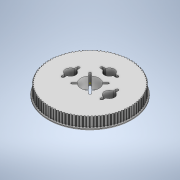
# Autodesk Inventor part: ZebatkaSilnik3
Saved by Autodesk Inventor 2021 (Build 250183000, 183)
## iProperties
Created: 2021-03-23
Part Number: ZebatkaSilnik3
Material: Ogólny
Document SubType Name: Modeling
Designer: micha
Density: 1 g/cm^3
Appearance: Domyślna
Author: micha
Autodesk Inventor part; units mm, degrees
(part 1 of 2)
ref_plane "YZ Plane" through (0, 0, 0) normal (1, 0, 0) x (0, 1, 0)
ref_plane "XZ Plane" through (0, 0, 0) normal (0, 1, 0) x (-1, 0, 0)
ref_plane "XY Plane" through (0, 0, 0) normal (0, 0, 1) x (1, 0, 0)
sketch "Szkic1" plane through (0, 0, 0) normal (0, 1, 0) x (-1, 0, 0)
  circle A0 centre (0, 0) radius 32.5
  dimension "d0" = 65
  constraints: 1 centre point, 1 coincident
  measures "d0" diameter of A0
extrude "Wyciągnięcie proste1" add sketch "Szkic1" along normal blind 1.5
sketch "Szkic3" plane through (0, 1.5, 0) normal (0, 1, 0) x (1, 0, 0)
  circle A0 centre (0, 0) radius 32.5 projected
  arc A1 (-30.7875, -0.0069) -> (-31.0611, 0.5149) centre (-31.3409, 0.0356) ccw
  arc A2 (-31.0611, 0.5149) -> (-31.3613, 0.6303) centre (-31.5652, -0.3487) ccw
  arc A3 (-31.4793, 0.7983) -> (-31.3613, 0.6303) centre (-31.3308, 0.7772) ccw
  line L0 (-32.4607, 1.0462) -> (-32.4793, 0.7969)
  line L1 (-31.4606, -1.0449) -> (-31.4793, -0.7955)
  arc A4 (-31.3613, -0.6278) -> (-31.4793, -0.7955) centre (-31.3307, -0.7746) ccw
  arc A5 (-31.061, -0.5126) -> (-30.7873, 0.0071) centre (-31.3409, -0.0332) ccw
  arc A6 (-31.3613, -0.6278) -> (-31.061, -0.5126) centre (-31.5647, 0.3513) ccw
  circle A7 centre (0, 0) radius 31.5
  line L2 (-31.4606, 1.0476) -> (-31.4793, 0.7983)
  line L3 (-31.3329, -3.0182) -> (-31.3672, -2.7706)
  arc A8 (-31.26, -2.5957) -> (-31.3672, -2.7706) centre (-31.2203, -2.7404) ccw
  arc A9 (-31.26, -2.5957) -> (-30.9676, -2.4619) centre (-31.5245, -1.6313) ccw
  arc A10 (-30.9676, -2.4619) -> (-30.727, -1.9261) centre (-31.2769, -2.0011) ccw
  arc A11 (-30.7263, -1.9401) -> (-31.0321, -1.4364) centre (-31.2813, -1.9323) ccw
  arc A12 (-31.0321, -1.4364) -> (-31.339, -1.3401) centre (-31.481, -2.33) ccw
  arc A13 (-31.4673, -1.1799) -> (-31.339, -1.3401) centre (-31.3177, -1.1916) ccw
  line L4 (-31.4643, -0.9299) -> (-31.4673, -1.1799)
  circle A14 centre (0, 0) radius 31.5
  line L5 (-31.0816, -4.9797) -> (-31.1313, -4.7347)
  arc A15 (-31.0354, -4.5534) -> (-31.1313, -4.7347) centre (-30.9866, -4.6953) ccw
  arc A16 (-31.0354, -4.5534) -> (-30.7519, -4.4015) centre (-31.3599, -3.6075) ccw
  arc A17 (-30.7519, -4.4015) -> (-30.5454, -3.8516) centre (-31.0896, -3.961) ccw
  arc A18 (-30.5439, -3.8656) -> (-30.8807, -3.3821) centre (-31.0982, -3.8927) ccw
  arc A19 (-30.8807, -3.3821) -> (-31.193, -3.3053) centre (-31.2726, -4.3021) ccw
  arc A20 (-31.3311, -3.1534) -> (-31.193, -3.3053) centre (-31.1811, -3.1557) ccw
  line L6 (-31.3438, -2.9037) -> (-31.3311, -3.1534)
  circle A21 centre (0, 0) radius 31.5
  line L7 (-30.7076, -6.9215) -> (-30.7726, -6.6801)
  arc A22 (-30.6882, -6.4932) -> (-30.7726, -6.6801) centre (-30.6306, -6.6317) ccw
  arc A23 (-30.6882, -6.4932) -> (-30.4148, -6.3237) centre (-31.0715, -5.5695) ccw
  arc A24 (-30.4148, -6.3237) -> (-30.2433, -5.762) centre (-30.7795, -5.9054) ccw
  arc A25 (-30.2409, -5.7758) -> (-30.6074, -5.3144) centre (-30.7924, -5.8377) ccw
  arc A26 (-30.6074, -5.3144) -> (-30.924, -5.2574) centre (-30.9408, -6.2572) ccw
  arc A27 (-31.0713, -5.1145) -> (-30.924, -5.2574) centre (-30.9214, -5.1074) ccw
  line L8 (-31.0996, -4.8661) -> (-31.0713, -5.1145)
  circle A28 centre (0, 0) radius 31.5
  line L9 (-30.2124, -8.836) -> (-30.2924, -8.5991)
  arc A29 (-30.2199, -8.4073) -> (-30.2924, -8.5991) centre (-30.1538, -8.5419) ccw
  arc A30 (-30.2199, -8.4073) -> (-29.9577, -8.221) centre (-30.6604, -7.5095) ccw
  arc A31 (-29.9577, -8.221) -> (-29.8219, -7.6496) centre (-30.348, -7.8264) ccw
  arc A32 (-29.8185, -7.6633) -> (-30.2133, -7.2258) centre (-30.3651, -7.7596) ccw
  arc A33 (-30.2133, -7.2258) -> (-30.5328, -7.1887) centre (-30.4868, -8.1877) ccw
  arc A34 (-30.6888, -7.0554) -> (-30.5328, -7.1887) centre (-30.5397, -7.0389) ccw
  line L10 (-30.7327, -6.8093) -> (-30.6888, -7.0554)
  circle A35 centre (0, 0) radius 31.5
  line L11 (-29.5979, -10.7156) -> (-29.6927, -10.4842)
  arc A36 (-29.6324, -10.2882) -> (-29.6927, -10.4842) centre (-29.5579, -10.4184) ccw
  arc A37 (-29.6324, -10.2882) -> (-29.3824, -10.0859) centre (-30.1284, -9.4199) ccw
  arc A38 (-29.3824, -10.0859) -> (-29.2827, -9.507) centre (-29.7966, -9.7165) ccw
  arc A39 (-29.2785, -9.5205) -> (-29.7, -9.1087) centre (-29.818, -9.651) ccw
  arc A40 (-29.7, -9.1087) -> (-30.0212, -9.0917) centre (-29.9126, -10.0858) ccw
  arc A41 (-30.1853, -8.9684) -> (-30.0212, -9.0917) centre (-30.0375, -8.9426) ccw
  line L12 (-30.2445, -8.7255) -> (-30.1853, -8.9684)
  circle A42 centre (0, 0) radius 31.5
  line L13 (-28.8667, -12.5529) -> (-28.9758, -12.328)
  arc A43 (-28.9279, -12.1285) -> (-28.9758, -12.328) centre (-28.8454, -12.2538) ccw
  arc A44 (-28.9279, -12.1285) -> (-28.6911, -11.9109) centre (-29.4775, -11.2931) ccw
  arc A45 (-28.6911, -11.9109) -> (-28.6279, -11.327) centre (-29.1277, -11.5683) ccw
  arc A46 (-28.623, -11.3401) -> (-29.0694, -10.9556) centre (-29.1531, -11.5042) ccw
  arc A47 (-29.0694, -10.9556) -> (-29.3911, -10.9588) centre (-29.2203, -11.9441) ccw
  arc A48 (-29.5626, -10.8461) -> (-29.3911, -10.9588) centre (-29.4167, -10.811) ccw
  line L14 (-29.637, -10.6074) -> (-29.5626, -10.8461)
  circle A49 centre (0, 0) radius 31.5
  line L15 (-28.0215, -14.3407) -> (-28.1446, -14.1231)
  arc A50 (-28.1093, -13.921) -> (-28.1446, -14.1231) centre (-28.0191, -14.0409) ccw
  arc A51 (-28.1093, -13.921) -> (-27.8866, -13.6889) centre (-28.7102, -13.1217) ccw
  arc A52 (-27.8866, -13.6889) -> (-27.8602, -13.1022) centre (-28.3439, -13.3744) ccw
  arc A53 (-27.8544, -13.115) -> (-28.3242, -12.7592) centre (-28.3732, -13.312) ccw
  arc A54 (-28.3242, -12.7592) -> (-28.645, -12.7827) centre (-28.4126, -13.7553) ccw
  arc A55 (-28.8232, -12.6809) -> (-28.645, -12.7827) centre (-28.6798, -12.6368) ccw
  line L16 (-28.9124, -12.4474) -> (-28.8232, -12.6809)
  circle A56 centre (0, 0) radius 31.5
  line L17 (-27.0658, -16.0719) -> (-27.2022, -15.8624)
  arc A57 (-27.1797, -15.6585) -> (-27.2022, -15.8624) centre (-27.0822, -15.7725) ccw
  arc A58 (-27.1797, -15.6585) -> (-26.9721, -15.4129) centre (-27.8296, -14.8985) ccw
  arc A59 (-26.9721, -15.4129) -> (-26.9826, -14.8257) centre (-27.4482, -15.1277) ccw
  arc A60 (-26.976, -14.8381) -> (-27.4671, -14.5125) centre (-27.4814, -15.0674) ccw
  arc A61 (-27.4671, -14.5125) -> (-27.7858, -14.5561) centre (-27.4928, -15.5122) ccw
  arc A62 (-27.9701, -14.4657) -> (-27.7858, -14.5561) centre (-27.8298, -14.4127) ccw
  line L18 (-28.0738, -14.2382) -> (-27.9701, -14.4657)
  circle A63 centre (0, 0) radius 31.5
  line L19 (-26.0032, -17.7396) -> (-26.1526, -17.5391)
  arc A64 (-26.1429, -17.3343) -> (-26.1526, -17.5391) centre (-26.0384, -17.4419) ccw
  arc A65 (-26.1429, -17.3343) -> (-25.9511, -17.0761) centre (-26.8392, -16.6166) ccw
  arc A66 (-25.9511, -17.0761) -> (-25.9984, -16.4907) centre (-26.4441, -16.8213) ccw
  arc A67 (-25.991, -16.5026) -> (-26.5017, -16.2086) centre (-26.4811, -16.7632) ccw
  arc A68 (-26.5017, -16.2086) -> (-26.817, -16.272) centre (-26.4646, -17.2079) ccw
  arc A69 (-27.0066, -16.1934) -> (-26.817, -16.272) centre (-26.8699, -16.1317) ccw
  line L20 (-27.1244, -15.9729) -> (-27.0066, -16.1934)
  circle A70 centre (0, 0) radius 31.5
  line L21 (-24.838, -19.3374) -> (-24.9997, -19.1467)
  arc A71 (-25.0029, -18.9416) -> (-24.9997, -19.1467) centre (-24.8918, -19.0424) ccw
  arc A72 (-25.0029, -18.9416) -> (-24.8276, -18.6719) centre (-25.7429, -18.269) ccw
  arc A73 (-24.8276, -18.6719) -> (-24.9117, -18.0906) centre (-25.3357, -18.4486) ccw
  arc A74 (-24.9035, -18.1021) -> (-25.4316, -17.8406) centre (-25.3763, -18.3929) ccw
  arc A75 (-25.4316, -17.8406) -> (-25.7424, -17.9238) centre (-25.3319, -18.8357) ccw
  arc A76 (-25.9365, -17.8572) -> (-25.7424, -17.9238) centre (-25.8039, -17.787) ccw
  line L22 (-26.0679, -17.6446) -> (-25.9365, -17.8572)
  circle A77 centre (0, 0) radius 31.5
  line L23 (-23.5748, -20.8588) -> (-23.7481, -20.6786)
  arc A78 (-23.7642, -20.4742) -> (-23.7481, -20.6786) centre (-23.647, -20.5678) ccw
  arc A79 (-23.7642, -20.4742) -> (-23.6062, -20.194) centre (-24.545, -19.8494) ccw
  arc A80 (-23.6062, -20.194) -> (-23.7266, -19.6191) centre (-24.1273, -20.003) ccw
  arc A81 (-23.7178, -19.6301) -> (-24.2612, -19.4023) centre (-24.1713, -19.95) ccw
  arc A82 (-24.2612, -19.4023) -> (-24.5661, -19.5048) centre (-24.0992, -20.3891) ccw
  arc A83 (-24.764, -19.4506) -> (-24.5661, -19.5048) centre (-24.6362, -19.3722) ccw
  line L24 (-24.9086, -19.2466) -> (-24.764, -19.4506)
  circle A84 centre (0, 0) radius 31.5
  line L25 (-22.2185, -22.2979) -> (-22.4028, -22.129)
  arc A85 (-22.4317, -21.9259) -> (-22.4028, -22.129) centre (-22.3089, -22.012) ccw
  arc A86 (-22.4317, -21.9259) -> (-22.2917, -21.6364) centre (-23.2502, -21.3514) ccw
  arc A87 (-22.2917, -21.6364) -> (-22.4479, -21.0702) centre (-22.8237, -21.4785) ccw
  arc A88 (-22.4384, -21.0806) -> (-22.9951, -20.8874) centre (-22.8709, -21.4283) ccw
  arc A89 (-22.9951, -20.8874) -> (-23.2929, -21.0088) centre (-22.7714, -21.8621) ccw
  arc A90 (-23.4939, -20.9671) -> (-23.2929, -21.0088) centre (-23.3712, -20.8808) ccw
  line L26 (-23.6509, -20.7726) -> (-23.4939, -20.9671)
  circle A91 centre (0, 0) radius 31.5
  line L27 (-20.7746, -23.649) -> (-20.9691, -23.492)
  arc A92 (-21.0107, -23.2912) -> (-20.9691, -23.492) centre (-20.8827, -23.3694) ccw
  arc A93 (-21.0107, -23.2912) -> (-20.8891, -22.9934) centre (-21.8637, -22.7692) ccw
  arc A94 (-20.8891, -22.9934) -> (-21.0806, -22.4381) centre (-21.4301, -22.8693) ccw
  arc A95 (-21.0704, -22.4479) -> (-21.6382, -22.29) centre (-21.4803, -22.8221) ccw
  arc A96 (-21.6382, -22.29) -> (-21.9278, -22.4299) centre (-21.3537, -23.2487) ccw
  arc A97 (-22.131, -22.4009) -> (-21.9278, -22.4299) centre (-22.0139, -22.3071) ccw
  line L28 (-22.2999, -22.2167) -> (-22.131, -22.4009)
  circle A98 centre (0, 0) radius 31.5
  line L29 (-19.2487, -24.9068) -> (-19.4527, -24.7623)
  arc A99 (-19.5068, -24.5645) -> (-19.4527, -24.7623) centre (-19.3741, -24.6345) ccw
  arc A100 (-19.5068, -24.5645) -> (-19.4041, -24.2597) centre (-20.3908, -24.0971) ccw
  arc A101 (-19.4041, -24.2597) -> (-19.6301, -23.7175) centre (-19.9518, -24.1697) ccw
  arc A102 (-19.6193, -23.7266) -> (-20.1958, -23.6047) centre (-20.0049, -24.1258) ccw
  arc A103 (-20.1958, -23.6047) -> (-20.4761, -23.7625) centre (-19.8518, -24.5437) ccw
  arc A104 (-20.6807, -23.7463) -> (-20.4761, -23.7625) centre (-20.5698, -23.6454) ccw
  line L30 (-20.8609, -23.573) -> (-20.6807, -23.7463)
  circle A105 centre (0, 0) radius 31.5
  line L31 (-17.6468, -26.0663) -> (-17.8594, -25.9349)
  arc A106 (-17.9259, -25.7408) -> (-17.8594, -25.9349) centre (-17.7891, -25.8024) ccw
  arc A107 (-17.9259, -25.7408) -> (-17.8426, -25.4302) centre (-18.8375, -25.3299) ccw
  arc A108 (-17.8426, -25.4302) -> (-18.1021, -24.9033) centre (-18.3948, -25.3748) ccw
  arc A109 (-18.0908, -24.9117) -> (-18.6738, -24.8263) centre (-18.4505, -25.3344) ccw
  arc A110 (-18.6738, -24.8263) -> (-18.9437, -25.0014) centre (-18.2715, -25.7417) ccw
  arc A111 (-19.1489, -24.998) -> (-18.9437, -25.0014) centre (-19.0445, -24.8903) ccw
  line L32 (-19.3396, -24.8364) -> (-19.1489, -24.998)
  circle A112 centre (0, 0) radius 31.5
  line L33 (-15.9752, -27.1229) -> (-16.1957, -27.0051)
  arc A113 (-16.2742, -26.8156) -> (-16.1957, -27.0051) centre (-16.1338, -26.8685) ccw
  arc A114 (-16.2742, -26.8156) -> (-16.2106, -26.5004) centre (-17.2099, -26.4627) ccw
  arc A115 (-16.2106, -26.5004) -> (-16.5027, -25.9908) centre (-16.7652, -26.4798) ccw
  arc A116 (-16.4909, -25.9985) -> (-17.0781, -25.9498) centre (-16.8234, -26.4429) ccw
  arc A117 (-17.0781, -25.9498) -> (-17.3364, -26.1415) centre (-16.6191, -26.8382) ccw
  arc A118 (-17.5415, -26.1511) -> (-17.3364, -26.1415) centre (-17.4441, -26.037) ccw
  line L34 (-17.7419, -26.0017) -> (-17.5415, -26.1511)
  circle A119 centre (0, 0) radius 31.5
  line L35 (-14.2406, -28.0725) -> (-14.4681, -27.9688)
  arc A120 (-14.5583, -27.7846) -> (-14.4681, -27.9688) centre (-14.4149, -27.8285) ccw
  arc A121 (-14.5583, -27.7846) -> (-14.5146, -27.4659) centre (-15.5143, -27.4911) ccw
  arc A122 (-14.5146, -27.4659) -> (-14.8381, -26.9757) centre (-15.0694, -27.4802) ccw
  arc A123 (-14.8259, -26.9826) -> (-15.415, -26.971) centre (-15.1298, -27.4471) ccw
  arc A124 (-15.415, -26.971) -> (-15.6608, -27.1785) centre (-14.9011, -27.8288) ccw
  arc A125 (-15.8648, -27.2009) -> (-15.6608, -27.1785) centre (-15.7748, -27.081) ccw
  line L36 (-16.0743, -27.0644) -> (-15.8648, -27.2009)
  circle A126 centre (0, 0) radius 31.5
  line L37 (-12.4499, -28.9113) -> (-12.6834, -28.822)
  arc A127 (-12.785, -28.6439) -> (-12.6834, -28.822) centre (-12.6391, -28.6787) ccw
  arc A128 (-12.785, -28.6439) -> (-12.7614, -28.3231) centre (-13.7575, -28.411) ccw
  arc A129 (-12.7614, -28.3231) -> (-13.115, -27.8542) centre (-13.3142, -28.3722) ccw
  arc A130 (-13.1024, -27.8603) -> (-13.6911, -27.8856) centre (-13.3765, -28.3429) ccw
  arc A131 (-13.6911, -27.8856) -> (-13.9233, -28.1082) centre (-13.1243, -28.7095) ccw
  arc A132 (-14.1255, -28.1434) -> (-13.9233, -28.1082) centre (-14.0432, -28.018) ccw
  line L38 (-14.3432, -28.0204) -> (-14.1255, -28.1434)
  circle A133 centre (0, 0) radius 31.5
  line L39 (-10.6099, -29.636) -> (-10.8486, -29.5615)
  arc A134 (-10.9612, -29.3901) -> (-10.8486, -29.5615) centre (-10.8134, -29.4157) ccw
  arc A135 (-10.9612, -29.3901) -> (-10.9578, -29.0685) centre (-11.9464, -29.2188) ccw
  arc A136 (-10.9578, -29.0685) -> (-11.3402, -28.6227) centre (-11.5064, -29.1522) ccw
  arc A137 (-11.3272, -28.6281) -> (-11.9131, -28.6903) centre (-11.5705, -29.1269) ccw
  arc A138 (-11.9131, -28.6903) -> (-12.1309, -28.927) centre (-11.2958, -29.477) ccw
  arc A139 (-12.3305, -28.9748) -> (-12.1309, -28.927) centre (-12.2562, -28.8445) ccw
  line L40 (-12.5554, -28.8657) -> (-12.3305, -28.9748)
  circle A140 centre (0, 0) radius 31.5
  line L41 (-8.7281, -30.2437) -> (-8.971, -30.1844)
  arc A141 (-9.0941, -30.0204) -> (-8.971, -30.1844) centre (-8.945, -30.0367) ccw
  arc A142 (-9.0941, -30.0204) -> (-9.1109, -29.6992) centre (-10.0882, -29.9113) ccw
  arc A143 (-9.1109, -29.6992) -> (-9.5206, -29.2783) centre (-9.6532, -29.8172) ccw
  arc A144 (-9.5073, -29.2828) -> (-10.0881, -29.3817) centre (-9.7188, -29.7959) ccw
  arc A145 (-10.0881, -29.3817) -> (-10.2907, -29.6316) centre (-9.4226, -30.1281) ccw
  arc A146 (-10.4869, -29.6919) -> (-10.2907, -29.6316) centre (-10.4209, -29.5572) ccw
  line L42 (-10.7182, -29.5971) -> (-10.4869, -29.6919)
  circle A147 centre (0, 0) radius 31.5
  line L43 (-6.8119, -30.732) -> (-7.058, -30.6881)
  arc A148 (-7.1912, -30.5322) -> (-7.058, -30.6881) centre (-7.0414, -30.5391) ccw
  arc A149 (-7.1912, -30.5322) -> (-7.2281, -30.2127) centre (-8.1901, -30.4857) ccw
  arc A150 (-7.2281, -30.2127) -> (-7.6634, -29.8183) centre (-7.7619, -30.3645) ccw
  arc A151 (-7.6498, -29.822) -> (-8.2233, -29.9572) centre (-7.8287, -30.3474) ccw
  arc A152 (-8.2233, -29.9572) -> (-8.4098, -30.2193) centre (-7.5122, -30.6603) ccw
  arc A153 (-8.6018, -30.2918) -> (-8.4098, -30.2193) centre (-8.5444, -30.1532) ccw
  line L44 (-8.8386, -30.2117) -> (-8.6018, -30.2918)
  circle A154 centre (0, 0) radius 31.5
  line L45 (-4.8688, -31.0991) -> (-5.1172, -31.0708)
  arc A155 (-5.2599, -30.9235) -> (-5.1172, -31.0708) centre (-5.1099, -30.9209) ccw
  arc A156 (-5.2599, -30.9235) -> (-5.3168, -30.6069) centre (-6.2598, -30.9398) ccw
  arc A157 (-5.3168, -30.6069) -> (-5.776, -30.2407) centre (-5.84, -30.792) ccw
  arc A158 (-5.7622, -30.2435) -> (-6.3261, -30.4144) centre (-5.9077, -30.7791) ccw
  arc A159 (-6.3261, -30.4144) -> (-6.4957, -30.6877) centre (-5.5722, -31.0715) ccw
  arc A160 (-6.6828, -30.7721) -> (-6.4957, -30.6877) centre (-6.6342, -30.6302) ccw
  line L46 (-6.9242, -30.707) -> (-6.6828, -30.7721)
  circle A161 centre (0, 0) radius 31.5
  line L47 (-2.9064, -31.3435) -> (-3.1561, -31.3308)
  arc A162 (-3.3078, -31.1927) -> (-3.1561, -31.3308) centre (-3.1583, -31.1808) ccw
  arc A163 (-3.3078, -31.1927) -> (-3.3845, -30.8804) centre (-4.3047, -31.2718) ccw
  arc A164 (-3.3845, -30.8804) -> (-3.8657, -30.5437) centre (-3.8951, -31.0979) ccw
  arc A165 (-3.8518, -30.5456) -> (-4.4039, -30.7516) centre (-3.9634, -31.0893) ccw
  arc A166 (-4.4039, -30.7516) -> (-4.556, -31.035) centre (-3.6103, -31.36) ccw
  arc A167 (-4.7374, -31.131) -> (-4.556, -31.035) centre (-4.6978, -30.9863) ccw
  line L48 (-4.9824, -31.0812) -> (-4.7374, -31.131)
  circle A168 centre (0, 0) radius 31.5
  line L49 (-0.9326, -31.4641) -> (-1.1826, -31.4671)
  arc A169 (-1.3427, -31.3389) -> (-1.1826, -31.4671) centre (-1.1942, -31.3176) ccw
  arc A170 (-1.3427, -31.3389) -> (-1.4388, -31.0319) centre (-2.3326, -31.4804) ccw
  arc A171 (-1.4388, -31.0319) -> (-1.9403, -30.7261) centre (-1.9347, -31.2811) ccw
  arc A172 (-1.9262, -30.7272) -> (-2.4643, -30.9675) centre (-2.0035, -31.2768) ccw
  arc A173 (-2.4643, -30.9675) -> (-2.5983, -31.2599) centre (-1.634, -31.5248) ccw
  arc A174 (-2.7733, -31.367) -> (-2.5983, -31.2599) centre (-2.7429, -31.2201) ccw
  line L50 (-3.021, -31.3327) -> (-2.7733, -31.367)
  circle A175 centre (0, 0) radius 31.5
  line L51 (1.0449, -31.4606) -> (0.7955, -31.4793)
  arc A176 (0.6278, -31.3613) -> (0.7955, -31.4793) centre (0.7746, -31.3307) ccw
  arc A177 (0.6278, -31.3613) -> (0.5126, -31.061) centre (-0.3513, -31.5647) ccw
  arc A178 (0.5126, -31.061) -> (-0.0071, -30.7873) centre (0.0332, -31.3409) ccw
  arc A179 (0.0069, -30.7875) -> (-0.5149, -31.0611) centre (-0.0356, -31.3409) ccw
  arc A180 (-0.5149, -31.0611) -> (-0.6303, -31.3613) centre (0.3487, -31.5652) ccw
  arc A181 (-0.7983, -31.4793) -> (-0.6303, -31.3613) centre (-0.7772, -31.3308) ccw
  line L52 (-1.0476, -31.4606) -> (-0.7983, -31.4793)
  circle A182 centre (0, 0) radius 31.5
  line L53 (3.0182, -31.3329) -> (2.7706, -31.3672)
  arc A183 (2.5957, -31.26) -> (2.7706, -31.3672) centre (2.7404, -31.2203) ccw
  arc A184 (2.5957, -31.26) -> (2.4619, -30.9676) centre (1.6313, -31.5245) ccw
  arc A185 (2.4619, -30.9676) -> (1.9261, -30.727) centre (2.0011, -31.2769) ccw
  arc A186 (1.9401, -30.7263) -> (1.4364, -31.0321) centre (1.9323, -31.2813) ccw
  arc A187 (1.4364, -31.0321) -> (1.3401, -31.339) centre (2.33, -31.481) ccw
  arc A188 (1.1799, -31.4673) -> (1.3401, -31.339) centre (1.1916, -31.3177) ccw
  line L54 (0.9299, -31.4643) -> (1.1799, -31.4673)
  circle A189 centre (0, 0) radius 31.5
  line L55 (4.9797, -31.0816) -> (4.7347, -31.1313)
  arc A190 (4.5534, -31.0354) -> (4.7347, -31.1313) centre (4.6953, -30.9866) ccw
  arc A191 (4.5534, -31.0354) -> (4.4015, -30.7519) centre (3.6075, -31.3599) ccw
  arc A192 (4.4015, -30.7519) -> (3.8516, -30.5454) centre (3.961, -31.0896) ccw
  arc A193 (3.8656, -30.5439) -> (3.3821, -30.8807) centre (3.8927, -31.0982) ccw
  arc A194 (3.3821, -30.8807) -> (3.3053, -31.193) centre (4.3021, -31.2726) ccw
  arc A195 (3.1534, -31.3311) -> (3.3053, -31.193) centre (3.1557, -31.1811) ccw
  line L56 (2.9037, -31.3438) -> (3.1534, -31.3311)
  circle A196 centre (0, 0) radius 31.5
  line L57 (6.9215, -30.7076) -> (6.6801, -30.7726)
  arc A197 (6.4932, -30.6882) -> (6.6801, -30.7726) centre (6.6317, -30.6306) ccw
  arc A198 (6.4932, -30.6882) -> (6.3237, -30.4148) centre (5.5695, -31.0715) ccw
  arc A199 (6.3237, -30.4148) -> (5.762, -30.2433) centre (5.9054, -30.7795) ccw
  arc A200 (5.7758, -30.2409) -> (5.3144, -30.6074) centre (5.8377, -30.7924) ccw
  arc A201 (5.3144, -30.6074) -> (5.2574, -30.924) centre (6.2572, -30.9408) ccw
  arc A202 (5.1145, -31.0713) -> (5.2574, -30.924) centre (5.1074, -30.9214) ccw
  line L58 (4.8661, -31.0996) -> (5.1145, -31.0713)
  circle A203 centre (0, 0) radius 31.5
  line L59 (8.836, -30.2124) -> (8.5991, -30.2924)
  arc A204 (8.4073, -30.2199) -> (8.5991, -30.2924) centre (8.5419, -30.1538) ccw
  arc A205 (8.4073, -30.2199) -> (8.221, -29.9577) centre (7.5095, -30.6604) ccw
  arc A206 (8.221, -29.9577) -> (7.6496, -29.8219) centre (7.8264, -30.348) ccw
  arc A207 (7.6633, -29.8185) -> (7.2258, -30.2133) centre (7.7596, -30.3651) ccw
  arc A208 (7.2258, -30.2133) -> (7.1887, -30.5328) centre (8.1877, -30.4868) ccw
  arc A209 (7.0554, -30.6888) -> (7.1887, -30.5328) centre (7.0389, -30.5397) ccw
  line L60 (6.8093, -30.7327) -> (7.0554, -30.6888)
  circle A210 centre (0, 0) radius 31.5
  line L61 (10.7156, -29.5979) -> (10.4842, -29.6927)
  arc A211 (10.2882, -29.6324) -> (10.4842, -29.6927) centre (10.4184, -29.5579) ccw
  arc A212 (10.2882, -29.6324) -> (10.0859, -29.3824) centre (9.4199, -30.1284) ccw
  arc A213 (10.0859, -29.3824) -> (9.507, -29.2827) centre (9.7165, -29.7966) ccw
  arc A214 (9.5205, -29.2785) -> (9.1087, -29.7) centre (9.651, -29.818) ccw
  arc A215 (9.1087, -29.7) -> (9.0917, -30.0212) centre (10.0858, -29.9126) ccw
  arc A216 (8.9684, -30.1853) -> (9.0917, -30.0212) centre (8.9426, -30.0375) ccw
  line L62 (8.7255, -30.2445) -> (8.9684, -30.1853)
  circle A217 centre (0, 0) radius 31.5
  line L63 (12.5529, -28.8667) -> (12.328, -28.9758)
  arc A218 (12.1285, -28.9279) -> (12.328, -28.9758) centre (12.2538, -28.8454) ccw
  arc A219 (12.1285, -28.9279) -> (11.9109, -28.6911) centre (11.2931, -29.4775) ccw
  arc A220 (11.9109, -28.6911) -> (11.327, -28.6279) centre (11.5683, -29.1277) ccw
  arc A221 (11.3401, -28.623) -> (10.9556, -29.0694) centre (11.5042, -29.1531) ccw
  arc A222 (10.9556, -29.0694) -> (10.9588, -29.3911) centre (11.9441, -29.2203) ccw
  arc A223 (10.8461, -29.5626) -> (10.9588, -29.3911) centre (10.811, -29.4167) ccw
  line L64 (10.6074, -29.637) -> (10.8461, -29.5626)
  circle A224 centre (0, 0) radius 31.5
  line L65 (14.3407, -28.0215) -> (14.1231, -28.1446)
  arc A225 (13.921, -28.1093) -> (14.1231, -28.1446) centre (14.0409, -28.0191) ccw
  arc A226 (13.921, -28.1093) -> (13.6889, -27.8866) centre (13.1217, -28.7102) ccw
  arc A227 (13.6889, -27.8866) -> (13.1022, -27.8602) centre (13.3744, -28.3439) ccw
  arc A228 (13.115, -27.8544) -> (12.7592, -28.3242) centre (13.312, -28.3732) ccw
  arc A229 (12.7592, -28.3242) -> (12.7827, -28.645) centre (13.7553, -28.4126) ccw
  arc A230 (12.6809, -28.8232) -> (12.7827, -28.645) centre (12.6368, -28.6798) ccw
  line L66 (12.4474, -28.9124) -> (12.6809, -28.8232)
  circle A231 centre (0, 0) radius 31.5
  line L67 (16.0719, -27.0658) -> (15.8624, -27.2022)
  arc A232 (15.6585, -27.1797) -> (15.8624, -27.2022) centre (15.7725, -27.0822) ccw
  arc A233 (15.6585, -27.1797) -> (15.4129, -26.9721) centre (14.8985, -27.8296) ccw
  arc A234 (15.4129, -26.9721) -> (14.8257, -26.9826) centre (15.1277, -27.4482) ccw
  arc A235 (14.8381, -26.976) -> (14.5125, -27.4671) centre (15.0674, -27.4814) ccw
  arc A236 (14.5125, -27.4671) -> (14.5561, -27.7858) centre (15.5122, -27.4928) ccw
  arc A237 (14.4657, -27.9701) -> (14.5561, -27.7858) centre (14.4127, -27.8298) ccw
  line L68 (14.2382, -28.0738) -> (14.4657, -27.9701)
  circle A238 centre (0, 0) radius 31.5
  line L69 (17.7396, -26.0032) -> (17.5391, -26.1526)
  arc A239 (17.3343, -26.1429) -> (17.5391, -26.1526) centre (17.4419, -26.0384) ccw
  arc A240 (17.3343, -26.1429) -> (17.0761, -25.9511) centre (16.6166, -26.8392) ccw
  arc A241 (17.0761, -25.9511) -> (16.4907, -25.9984) centre (16.8213, -26.4441) ccw
  arc A242 (16.5026, -25.991) -> (16.2086, -26.5017) centre (16.7632, -26.4811) ccw
  arc A243 (16.2086, -26.5017) -> (16.272, -26.817) centre (17.2079, -26.4646) ccw
  arc A244 (16.1934, -27.0066) -> (16.272, -26.817) centre (16.1317, -26.8699) ccw
  line L70 (15.9729, -27.1244) -> (16.1934, -27.0066)
  circle A245 centre (0, 0) radius 31.5
  line L71 (19.3374, -24.838) -> (19.1467, -24.9997)
  arc A246 (18.9416, -25.0029) -> (19.1467, -24.9997) centre (19.0424, -24.8918) ccw
  arc A247 (18.9416, -25.0029) -> (18.6719, -24.8276) centre (18.269, -25.7429) ccw
  arc A248 (18.6719, -24.8276) -> (18.0906, -24.9117) centre (18.4486, -25.3357) ccw
  arc A249 (18.1021, -24.9035) -> (17.8406, -25.4316) centre (18.3929, -25.3763) ccw
  arc A250 (17.8406, -25.4316) -> (17.9238, -25.7424) centre (18.8357, -25.3319) ccw
  arc A251 (17.8572, -25.9365) -> (17.9238, -25.7424) centre (17.787, -25.8039) ccw
  line L72 (17.6446, -26.0679) -> (17.8572, -25.9365)
  circle A252 centre (0, 0) radius 31.5
  line L73 (20.8588, -23.5748) -> (20.6786, -23.7481)
  arc A253 (20.4742, -23.7642) -> (20.6786, -23.7481) centre (20.5678, -23.647) ccw
  arc A254 (20.4742, -23.7642) -> (20.194, -23.6062) centre (19.8494, -24.545) ccw
  arc A255 (20.194, -23.6062) -> (19.6191, -23.7266) centre (20.003, -24.1273) ccw
  arc A256 (19.6301, -23.7178) -> (19.4023, -24.2612) centre (19.95, -24.1713) ccw
  arc A257 (19.4023, -24.2612) -> (19.5048, -24.5661) centre (20.3891, -24.0992) ccw
  arc A258 (19.4506, -24.764) -> (19.5048, -24.5661) centre (19.3722, -24.6362) ccw
  line L74 (19.2466, -24.9086) -> (19.4506, -24.764)
  circle A259 centre (0, 0) radius 31.5
  line L75 (22.2979, -22.2185) -> (22.129, -22.4028)
  arc A260 (21.9259, -22.4317) -> (22.129, -22.4028) centre (22.012, -22.3089) ccw
  arc A261 (21.9259, -22.4317) -> (21.6364, -22.2917) centre (21.3514, -23.2502) ccw
  arc A262 (21.6364, -22.2917) -> (21.0702, -22.4479) centre (21.4785, -22.8237) ccw
  arc A263 (21.0806, -22.4384) -> (20.8874, -22.9951) centre (21.4283, -22.8709) ccw
  arc A264 (20.8874, -22.9951) -> (21.0088, -23.2929) centre (21.8621, -22.7714) ccw
  arc A265 (20.9671, -23.4939) -> (21.0088, -23.2929) centre (20.8808, -23.3712) ccw
  line L76 (20.7726, -23.6509) -> (20.9671, -23.4939)
  circle A266 centre (0, 0) radius 31.5
  line L77 (23.649, -20.7746) -> (23.492, -20.9691)
  arc A267 (23.2912, -21.0107) -> (23.492, -20.9691) centre (23.3694, -20.8827) ccw
  arc A268 (23.2912, -21.0107) -> (22.9934, -20.8891) centre (22.7692, -21.8637) ccw
  arc A269 (22.9934, -20.8891) -> (22.4381, -21.0806) centre (22.8693, -21.4301) ccw
  arc A270 (22.4479, -21.0704) -> (22.29, -21.6382) centre (22.8221, -21.4803) ccw
  arc A271 (22.29, -21.6382) -> (22.4299, -21.9278) centre (23.2487, -21.3537) ccw
  arc A272 (22.4009, -22.131) -> (22.4299, -21.9278) centre (22.3071, -22.0139) ccw
  line L78 (22.2167, -22.2999) -> (22.4009, -22.131)
  circle A273 centre (0, 0) radius 31.5
  line L79 (24.9068, -19.2487) -> (24.7623, -19.4527)
  arc A274 (24.5645, -19.5068) -> (24.7623, -19.4527) centre (24.6345, -19.3741) ccw
  arc A275 (24.5645, -19.5068) -> (24.2597, -19.4041) centre (24.0971, -20.3908) ccw
  arc A276 (24.2597, -19.4041) -> (23.7175, -19.6301) centre (24.1697, -19.9518) ccw
  arc A277 (23.7266, -19.6193) -> (23.6047, -20.1958) centre (24.1258, -20.0049) ccw
  arc A278 (23.6047, -20.1958) -> (23.7625, -20.4761) centre (24.5437, -19.8518) ccw
  arc A279 (23.7463, -20.6807) -> (23.7625, -20.4761) centre (23.6454, -20.5698) ccw
  line L80 (23.573, -20.8609) -> (23.7463, -20.6807)
  circle A280 centre (0, 0) radius 31.5
  line L81 (26.0663, -17.6468) -> (25.9349, -17.8594)
  arc A281 (25.7408, -17.9259) -> (25.9349, -17.8594) centre (25.8024, -17.7891) ccw
  arc A282 (25.7408, -17.9259) -> (25.4302, -17.8426) centre (25.3299, -18.8375) ccw
  arc A283 (25.4302, -17.8426) -> (24.9033, -18.1021) centre (25.3748, -18.3948) ccw
  arc A284 (24.9117, -18.0908) -> (24.8263, -18.6738) centre (25.3344, -18.4505) ccw
  arc A285 (24.8263, -18.6738) -> (25.0014, -18.9437) centre (25.7417, -18.2715) ccw
  arc A286 (24.998, -19.1489) -> (25.0014, -18.9437) centre (24.8903, -19.0445) ccw
  line L82 (24.8364, -19.3396) -> (24.998, -19.1489)
  circle A287 centre (0, 0) radius 31.5
  line L83 (27.1229, -15.9752) -> (27.0051, -16.1957)
  arc A288 (26.8156, -16.2742) -> (27.0051, -16.1957) centre (26.8685, -16.1338) ccw
  arc A289 (26.8156, -16.2742) -> (26.5004, -16.2106) centre (26.4627, -17.2099) ccw
  arc A290 (26.5004, -16.2106) -> (25.9908, -16.5027) centre (26.4798, -16.7652) ccw
  arc A291 (25.9985, -16.4909) -> (25.9498, -17.0781) centre (26.4429, -16.8234) ccw
  arc A292 (25.9498, -17.0781) -> (26.1415, -17.3364) centre (26.8382, -16.6191) ccw
  arc A293 (26.1511, -17.5415) -> (26.1415, -17.3364) centre (26.037, -17.4441) ccw
  line L84 (26.0017, -17.7419) -> (26.1511, -17.5415)
  circle A294 centre (0, 0) radius 31.5
  line L85 (28.0725, -14.2406) -> (27.9688, -14.4681)
  arc A295 (27.7846, -14.5583) -> (27.9688, -14.4681) centre (27.8285, -14.4149) ccw
  arc A296 (27.7846, -14.5583) -> (27.4659, -14.5146) centre (27.4911, -15.5143) ccw
  arc A297 (27.4659, -14.5146) -> (26.9757, -14.8381) centre (27.4802, -15.0694) ccw
  arc A298 (26.9826, -14.8259) -> (26.971, -15.415) centre (27.4471, -15.1298) ccw
  arc A299 (26.971, -15.415) -> (27.1785, -15.6608) centre (27.8288, -14.9011) ccw
  arc A300 (27.2009, -15.8648) -> (27.1785, -15.6608) centre (27.081, -15.7748) ccw
  line L86 (27.0644, -16.0743) -> (27.2009, -15.8648)
  circle A301 centre (0, 0) radius 31.5
  line L87 (28.9113, -12.4499) -> (28.822, -12.6834)
  arc A302 (28.6439, -12.785) -> (28.822, -12.6834) centre (28.6787, -12.6391) ccw
  arc A303 (28.6439, -12.785) -> (28.3231, -12.7614) centre (28.411, -13.7575) ccw
  arc A304 (28.3231, -12.7614) -> (27.8542, -13.115) centre (28.3722, -13.3142) ccw
  arc A305 (27.8603, -13.1024) -> (27.8856, -13.6911) centre (28.3429, -13.3765) ccw
  arc A306 (27.8856, -13.6911) -> (28.1082, -13.9233) centre (28.7095, -13.1243) ccw
  arc A307 (28.1434, -14.1255) -> (28.1082, -13.9233) centre (28.018, -14.0432) ccw
  line L88 (28.0204, -14.3432) -> (28.1434, -14.1255)
  circle A308 centre (0, 0) radius 31.5
  line L89 (29.636, -10.6099) -> (29.5615, -10.8486)
  arc A309 (29.3901, -10.9612) -> (29.5615, -10.8486) centre (29.4157, -10.8134) ccw
  arc A310 (29.3901, -10.9612) -> (29.0685, -10.9578) centre (29.2188, -11.9464) ccw
  arc A311 (29.0685, -10.9578) -> (28.6227, -11.3402) centre (29.1522, -11.5064) ccw
  arc A312 (28.6281, -11.3272) -> (28.6903, -11.9131) centre (29.1269, -11.5705) ccw
  arc A313 (28.6903, -11.9131) -> (28.927, -12.1309) centre (29.477, -11.2958) ccw
  arc A314 (28.9748, -12.3305) -> (28.927, -12.1309) centre (28.8445, -12.2562) ccw
  line L90 (28.8657, -12.5554) -> (28.9748, -12.3305)
  circle A315 centre (0, 0) radius 31.5
  line L91 (30.2437, -8.7281) -> (30.1844, -8.971)
  arc A316 (30.0204, -9.0941) -> (30.1844, -8.971) centre (30.0367, -8.945) ccw
  arc A317 (30.0204, -9.0941) -> (29.6992, -9.1109) centre (29.9113, -10.0882) ccw
  arc A318 (29.6992, -9.1109) -> (29.2783, -9.5206) centre (29.8172, -9.6532) ccw
  arc A319 (29.2828, -9.5073) -> (29.3817, -10.0881) centre (29.7959, -9.7188) ccw
  arc A320 (29.3817, -10.0881) -> (29.6316, -10.2907) centre (30.1281, -9.4226) ccw
  arc A321 (29.6919, -10.4869) -> (29.6316, -10.2907) centre (29.5572, -10.4209) ccw
  line L92 (29.5971, -10.7182) -> (29.6919, -10.4869)
  circle A322 centre (0, 0) radius 31.5
  line L93 (30.732, -6.8119) -> (30.6881, -7.058)
  arc A323 (30.5322, -7.1912) -> (30.6881, -7.058) centre (30.5391, -7.0414) ccw
  arc A324 (30.5322, -7.1912) -> (30.2127, -7.2281) centre (30.4857, -8.1901) ccw
  arc A325 (30.2127, -7.2281) -> (29.8183, -7.6634) centre (30.3645, -7.7619) ccw
  arc A326 (29.822, -7.6498) -> (29.9572, -8.2233) centre (30.3474, -7.8287) ccw
  arc A327 (29.9572, -8.2233) -> (30.2193, -8.4098) centre (30.6603, -7.5122) ccw
  arc A328 (30.2918, -8.6018) -> (30.2193, -8.4098) centre (30.1532, -8.5444) ccw
  line L94 (30.2117, -8.8386) -> (30.2918, -8.6018)
  circle A329 centre (0, 0) radius 31.5
  line L95 (31.0991, -4.8688) -> (31.0708, -5.1172)
  arc A330 (30.9235, -5.2599) -> (31.0708, -5.1172) centre (30.9209, -5.1099) ccw
  arc A331 (30.9235, -5.2599) -> (30.6069, -5.3168) centre (30.9398, -6.2598) ccw
  arc A332 (30.6069, -5.3168) -> (30.2407, -5.776) centre (30.792, -5.84) ccw
  arc A333 (30.2435, -5.7622) -> (30.4144, -6.3261) centre (30.7791, -5.9077) ccw
  arc A334 (30.4144, -6.3261) -> (30.6877, -6.4957) centre (31.0715, -5.5722) ccw
  arc A335 (30.7721, -6.6828) -> (30.6877, -6.4957) centre (30.6302, -6.6342) ccw
  line L96 (30.707, -6.9242) -> (30.7721, -6.6828)
  circle A336 centre (0, 0) radius 31.5
  line L97 (31.3435, -2.9064) -> (31.3308, -3.1561)
  arc A337 (31.1927, -3.3078) -> (31.3308, -3.1561) centre (31.1808, -3.1583) ccw
  arc A338 (31.1927, -3.3078) -> (30.8804, -3.3845) centre (31.2718, -4.3047) ccw
  arc A339 (30.8804, -3.3845) -> (30.5437, -3.8657) centre (31.0979, -3.8951) ccw
  arc A340 (30.5456, -3.8518) -> (30.7516, -4.4039) centre (31.0893, -3.9634) ccw
  arc A341 (30.7516, -4.4039) -> (31.035, -4.556) centre (31.36, -3.6103) ccw
  arc A342 (31.131, -4.7374) -> (31.035, -4.556) centre (30.9863, -4.6978) ccw
  line L98 (31.0812, -4.9824) -> (31.131, -4.7374)
  circle A343 centre (0, 0) radius 31.5
  line L99 (31.4641, -0.9326) -> (31.4671, -1.1826)
  arc A344 (31.3389, -1.3427) -> (31.4671, -1.1826) centre (31.3176, -1.1942) ccw
  arc A345 (31.3389, -1.3427) -> (31.0319, -1.4388) centre (31.4804, -2.3326) ccw
  arc A346 (31.0319, -1.4388) -> (30.7261, -1.9403) centre (31.2811, -1.9347) ccw
  arc A347 (30.7272, -1.9262) -> (30.9675, -2.4643) centre (31.2768, -2.0035) ccw
  arc A348 (30.9675, -2.4643) -> (31.2599, -2.5983) centre (31.5248, -1.634) ccw
  arc A349 (31.367, -2.7733) -> (31.2599, -2.5983) centre (31.2201, -2.7429) ccw
  line L100 (31.3327, -3.021) -> (31.367, -2.7733)
  circle A350 centre (0, 0) radius 31.5
  line L101 (31.4606, 1.0449) -> (31.4793, 0.7955)
  arc A351 (31.3613, 0.6278) -> (31.4793, 0.7955) centre (31.3307, 0.7746) ccw
  arc A352 (31.3613, 0.6278) -> (31.061, 0.5126) centre (31.5647, -0.3513) ccw
  arc A353 (31.061, 0.5126) -> (30.7873, -0.0071) centre (31.3409, 0.0332) ccw
  arc A354 (30.7875, 0.0069) -> (31.0611, -0.5149) centre (31.3409, -0.0356) ccw
  arc A355 (31.0611, -0.5149) -> (31.3613, -0.6303) centre (31.5652, 0.3487) ccw
  arc A356 (31.4793, -0.7983) -> (31.3613, -0.6303) centre (31.3308, -0.7772) ccw
  line L102 (31.4606, -1.0476) -> (31.4793, -0.7983)
  circle A357 centre (0, 0) radius 31.5
  line L103 (31.3329, 3.0182) -> (31.3672, 2.7706)
  arc A358 (31.26, 2.5957) -> (31.3672, 2.7706) centre (31.2203, 2.7404) ccw
  arc A359 (31.26, 2.5957) -> (30.9676, 2.4619) centre (31.5245, 1.6313) ccw
  arc A360 (30.9676, 2.4619) -> (30.727, 1.9261) centre (31.2769, 2.0011) ccw
  arc A361 (30.7263, 1.9401) -> (31.0321, 1.4364) centre (31.2813, 1.9323) ccw
  arc A362 (31.0321, 1.4364) -> (31.339, 1.3401) centre (31.481, 2.33) ccw
  arc A363 (31.4673, 1.1799) -> (31.339, 1.3401) centre (31.3177, 1.1916) ccw
  line L104 (31.4643, 0.9299) -> (31.4673, 1.1799)
  circle A364 centre (0, 0) radius 31.5
  line L105 (31.0816, 4.9797) -> (31.1313, 4.7347)
  arc A365 (31.0354, 4.5534) -> (31.1313, 4.7347) centre (30.9866, 4.6953) ccw
  arc A366 (31.0354, 4.5534) -> (30.7519, 4.4015) centre (31.3599, 3.6075) ccw
  arc A367 (30.7519, 4.4015) -> (30.5454, 3.8516) centre (31.0896, 3.961) ccw
  arc A368 (30.5439, 3.8656) -> (30.8807, 3.3821) centre (31.0982, 3.8927) ccw
  arc A369 (30.8807, 3.3821) -> (31.193, 3.3053) centre (31.2726, 4.3021) ccw
  arc A370 (31.3311, 3.1534) -> (31.193, 3.3053) centre (31.1811, 3.1557) ccw
  line L106 (31.3438, 2.9037) -> (31.3311, 3.1534)
  circle A371 centre (0, 0) radius 31.5
  line L107 (30.7076, 6.9215) -> (30.7726, 6.6801)
  arc A372 (30.6882, 6.4932) -> (30.7726, 6.6801) centre (30.6306, 6.6317) ccw
  arc A373 (30.6882, 6.4932) -> (30.4148, 6.3237) centre (31.0715, 5.5695) ccw
  arc A374 (30.4148, 6.3237) -> (30.2433, 5.762) centre (30.7795, 5.9054) ccw
  arc A375 (30.2409, 5.7758) -> (30.6074, 5.3144) centre (30.7924, 5.8377) ccw
  arc A376 (30.6074, 5.3144) -> (30.924, 5.2574) centre (30.9408, 6.2572) ccw
  arc A377 (31.0713, 5.1145) -> (30.924, 5.2574) centre (30.9214, 5.1074) ccw
  line L108 (31.0996, 4.8661) -> (31.0713, 5.1145)
  circle A378 centre (0, 0) radius 31.5
  line L109 (30.2124, 8.836) -> (30.2924, 8.5991)
  arc A379 (30.2199, 8.4073) -> (30.2924, 8.5991) centre (30.1538, 8.5419) ccw
  arc A380 (30.2199, 8.4073) -> (29.9577, 8.221) centre (30.6604, 7.5095) ccw
  arc A381 (29.9577, 8.221) -> (29.8219, 7.6496) centre (30.348, 7.8264) ccw
  arc A382 (29.8185, 7.6633) -> (30.2133, 7.2258) centre (30.3651, 7.7596) ccw
  arc A383 (30.2133, 7.2258) -> (30.5328, 7.1887) centre (30.4868, 8.1877) ccw
  arc A384 (30.6888, 7.0554) -> (30.5328, 7.1887) centre (30.5397, 7.0389) ccw
  line L110 (30.7327, 6.8093) -> (30.6888, 7.0554)
  circle A385 centre (0, 0) radius 31.5
  line L111 (29.5979, 10.7156) -> (29.6927, 10.4842)
  arc A386 (29.6324, 10.2882) -> (29.6927, 10.4842) centre (29.5579, 10.4184) ccw
  arc A387 (29.6324, 10.2882) -> (29.3824, 10.0859) centre (30.1284, 9.4199) ccw
  arc A388 (29.3824, 10.0859) -> (29.2827, 9.507) centre (29.7966, 9.7165) ccw
  arc A389 (29.2785, 9.5205) -> (29.7, 9.1087) centre (29.818, 9.651) ccw
  arc A390 (29.7, 9.1087) -> (30.0212, 9.0917) centre (29.9126, 10.0858) ccw
  arc A391 (30.1853, 8.9684) -> (30.0212, 9.0917) centre (30.0375, 8.9426) ccw
  line L112 (30.2445, 8.7255) -> (30.1853, 8.9684)
  circle A392 centre (0, 0) radius 31.5
  line L113 (28.8667, 12.5529) -> (28.9758, 12.328)
  arc A393 (28.9279, 12.1285) -> (28.9758, 12.328) centre (28.8454, 12.2538) ccw
  arc A394 (28.9279, 12.1285) -> (28.6911, 11.9109) centre (29.4775, 11.2931) ccw
  arc A395 (28.6911, 11.9109) -> (28.6279, 11.327) centre (29.1277, 11.5683) ccw
  arc A396 (28.623, 11.3401) -> (29.0694, 10.9556) centre (29.1531, 11.5042) ccw
  arc A397 (29.0694, 10.9556) -> (29.3911, 10.9588) centre (29.2203, 11.9441) ccw
  arc A398 (29.5626, 10.8461) -> (29.3911, 10.9588) centre (29.4167, 10.811) ccw
  line L114 (29.637, 10.6074) -> (29.5626, 10.8461)
  circle A399 centre (0, 0) radius 31.5
  line L115 (28.0215, 14.3407) -> (28.1446, 14.1231)
  arc A400 (28.1093, 13.921) -> (28.1446, 14.1231) centre (28.0191, 14.0409) ccw
  arc A401 (28.1093, 13.921) -> (27.8866, 13.6889) centre (28.7102, 13.1217) ccw
  arc A402 (27.8866, 13.6889) -> (27.8602, 13.1022) centre (28.3439, 13.3744) ccw
  arc A403 (27.8544, 13.115) -> (28.3242, 12.7592) centre (28.3732, 13.312) ccw
  arc A404 (28.3242, 12.7592) -> (28.645, 12.7827) centre (28.4126, 13.7553) ccw
  arc A405 (28.8232, 12.6809) -> (28.645, 12.7827) centre (28.6798, 12.6368) ccw
  line L116 (28.9124, 12.4474) -> (28.8232, 12.6809)
  circle A406 centre (0, 0) radius 31.5
  line L117 (27.0658, 16.0719) -> (27.2022, 15.8624)
  arc A407 (27.1797, 15.6585) -> (27.2022, 15.8624) centre (27.0822, 15.7725) ccw
  arc A408 (27.1797, 15.6585) -> (26.9721, 15.4129) centre (27.8296, 14.8985) ccw
  arc A409 (26.9721, 15.4129) -> (26.9826, 14.8257) centre (27.4482, 15.1277) ccw
  arc A410 (26.976, 14.8381) -> (27.4671, 14.5125) centre (27.4814, 15.0674) ccw
  arc A411 (27.4671, 14.5125) -> (27.7858, 14.5561) centre (27.4928, 15.5122) ccw
  arc A412 (27.9701, 14.4657) -> (27.7858, 14.5561) centre (27.8298, 14.4127) ccw
  line L118 (28.0738, 14.2382) -> (27.9701, 14.4657)
  circle A413 centre (0, 0) radius 31.5
  line L119 (26.0032, 17.7396) -> (26.1526, 17.5391)
  arc A414 (26.1429, 17.3343) -> (26.1526, 17.5391) centre (26.0384, 17.4419) ccw
  arc A415 (26.1429, 17.3343) -> (25.9511, 17.0761) centre (26.8392, 16.6166) ccw
  arc A416 (25.9511, 17.0761) -> (25.9984, 16.4907) centre (26.4441, 16.8213) ccw
  arc A417 (25.991, 16.5026) -> (26.5017, 16.2086) centre (26.4811, 16.7632) ccw
  arc A418 (26.5017, 16.2086) -> (26.817, 16.272) centre (26.4646, 17.2079) ccw
  arc A419 (27.0066, 16.1934) -> (26.817, 16.272) centre (26.8699, 16.1317) ccw
  line L120 (27.1244, 15.9729) -> (27.0066, 16.1934)
  circle A420 centre (0, 0) radius 31.5
  line L121 (24.838, 19.3374) -> (24.9997, 19.1467)
  arc A421 (25.0029, 18.9416) -> (24.9997, 19.1467) centre (24.8918, 19.0424) ccw
  arc A422 (25.0029, 18.9416) -> (24.8276, 18.6719) centre (25.7429, 18.269) ccw
  arc A423 (24.8276, 18.6719) -> (24.9117, 18.0906) centre (25.3357, 18.4486) ccw
  arc A424 (24.9035, 18.1021) -> (25.4316, 17.8406) centre (25.3763, 18.3929) ccw
  arc A425 (25.4316, 17.8406) -> (25.7424, 17.9238) centre (25.3319, 18.8357) ccw
  arc A426 (25.9365, 17.8572) -> (25.7424, 17.9238) centre (25.8039, 17.787) ccw
  line L122 (26.0679, 17.6446) -> (25.9365, 17.8572)
  circle A427 centre (0, 0) radius 31.5
  line L123 (23.5748, 20.8588) -> (23.7481, 20.6786)
  arc A428 (23.7642, 20.4742) -> (23.7481, 20.6786) centre (23.647, 20.5678) ccw
  arc A429 (23.7642, 20.4742) -> (23.6062, 20.194) centre (24.545, 19.8494) ccw
  arc A430 (23.6062, 20.194) -> (23.7266, 19.6191) centre (24.1273, 20.003) ccw
  arc A431 (23.7178, 19.6301) -> (24.2612, 19.4023) centre (24.1713, 19.95) ccw
  arc A432 (24.2612, 19.4023) -> (24.5661, 19.5048) centre (24.0992, 20.3891) ccw
  arc A433 (24.764, 19.4506) -> (24.5661, 19.5048) centre (24.6362, 19.3722) ccw
  line L124 (24.9086, 19.2466) -> (24.764, 19.4506)
  circle A434 centre (0, 0) radius 31.5
  line L125 (22.2185, 22.2979) -> (22.4028, 22.129)
  arc A435 (22.4317, 21.9259) -> (22.4028, 22.129) centre (22.3089, 22.012) ccw
  arc A436 (22.4317, 21.9259) -> (22.2917, 21.6364) centre (23.2502, 21.3514) ccw
  arc A437 (22.2917, 21.6364) -> (22.4479, 21.0702) centre (22.8237, 21.4785) ccw
  arc A438 (22.4384, 21.0806) -> (22.9951, 20.8874) centre (22.8709, 21.4283) ccw
  arc A439 (22.9951, 20.8874) -> (23.2929, 21.0088) centre (22.7714, 21.8621) ccw
  arc A440 (23.4939, 20.9671) -> (23.2929, 21.0088) centre (23.3712, 20.8808) ccw
  line L126 (23.6509, 20.7726) -> (23.4939, 20.9671)
  circle A441 centre (0, 0) radius 31.5
  line L127 (20.7746, 23.649) -> (20.9691, 23.492)
  arc A442 (21.0107, 23.2912) -> (20.9691, 23.492) centre (20.8827, 23.3694) ccw
  arc A443 (21.0107, 23.2912) -> (20.8891, 22.9934) centre (21.8637, 22.7692) ccw
  arc A444 (20.8891, 22.9934) -> (21.0806, 22.4381) centre (21.4301, 22.8693) ccw
  arc A445 (21.0704, 22.4479) -> (21.6382, 22.29) centre (21.4803, 22.8221) ccw
  arc A446 (21.6382, 22.29) -> (21.9278, 22.4299) centre (21.3537, 23.2487) ccw
  arc A447 (22.131, 22.4009) -> (21.9278, 22.4299) centre (22.0139, 22.3071) ccw
  line L128 (22.2999, 22.2167) -> (22.131, 22.4009)
  circle A448 centre (0, 0) radius 31.5
  line L129 (19.2487, 24.9068) -> (19.4527, 24.7623)
  arc A449 (19.5068, 24.5645) -> (19.4527, 24.7623) centre (19.3741, 24.6345) ccw
  arc A450 (19.5068, 24.5645) -> (19.4041, 24.2597) centre (20.3908, 24.0971) ccw
  arc A451 (19.4041, 24.2597) -> (19.6301, 23.7175) centre (19.9518, 24.1697) ccw
  arc A452 (19.6193, 23.7266) -> (20.1958, 23.6047) centre (20.0049, 24.1258) ccw
  arc A453 (20.1958, 23.6047) -> (20.4761, 23.7625) centre (19.8518, 24.5437) ccw
  arc A454 (20.6807, 23.7463) -> (20.4761, 23.7625) centre (20.5698, 23.6454) ccw
  line L130 (20.8609, 23.573) -> (20.6807, 23.7463)
  circle A455 centre (0, 0) radius 31.5
  line L131 (17.6468, 26.0663) -> (17.8594, 25.9349)
  arc A456 (17.9259, 25.7408) -> (17.8594, 25.9349) centre (17.7891, 25.8024) ccw
  arc A457 (17.9259, 25.7408) -> (17.8426, 25.4302) centre (18.8375, 25.3299) ccw
  arc A458 (17.8426, 25.4302) -> (18.1021, 24.9033) centre (18.3948, 25.3748) ccw
  arc A459 (18.0908, 24.9117) -> (18.6738, 24.8263) centre (18.4505, 25.3344) ccw
  arc A460 (18.6738, 24.8263) -> (18.9437, 25.0014) centre (18.2715, 25.7417) ccw
  arc A461 (19.1489, 24.998) -> (18.9437, 25.0014) centre (19.0445, 24.8903) ccw
  line L132 (19.3396, 24.8364) -> (19.1489, 24.998)
  circle A462 centre (0, 0) radius 31.5
  line L133 (15.9752, 27.1229) -> (16.1957, 27.0051)
  arc A463 (16.2742, 26.8156) -> (16.1957, 27.0051) centre (16.1338, 26.8685) ccw
  arc A464 (16.2742, 26.8156) -> (16.2106, 26.5004) centre (17.2099, 26.4627) ccw
  arc A465 (16.2106, 26.5004) -> (16.5027, 25.9908) centre (16.7652, 26.4798) ccw
  arc A466 (16.4909, 25.9985) -> (17.0781, 25.9498) centre (16.8234, 26.4429) ccw
  arc A467 (17.0781, 25.9498) -> (17.3364, 26.1415) centre (16.6191, 26.8382) ccw
  arc A468 (17.5415, 26.1511) -> (17.3364, 26.1415) centre (17.4441, 26.037) ccw
  line L134 (17.7419, 26.0017) -> (17.5415, 26.1511)
  circle A469 centre (0, 0) radius 31.5
  line L135 (14.2406, 28.0725) -> (14.4681, 27.9688)
  arc A470 (14.5583, 27.7846) -> (14.4681, 27.9688) centre (14.4149, 27.8285) ccw
  arc A471 (14.5583, 27.7846) -> (14.5146, 27.4659) centre (15.5143, 27.4911) ccw
  arc A472 (14.5146, 27.4659) -> (14.8381, 26.9757) centre (15.0694, 27.4802) ccw
  arc A473 (14.8259, 26.9826) -> (15.415, 26.971) centre (15.1298, 27.4471) ccw
  arc A474 (15.415, 26.971) -> (15.6608, 27.1785) centre (14.9011, 27.8288) ccw
  arc A475 (15.8648, 27.2009) -> (15.6608, 27.1785) centre (15.7748, 27.081) ccw
  line L136 (16.0743, 27.0644) -> (15.8648, 27.2009)
  circle A476 centre (0, 0) radius 31.5
  line L137 (12.4499, 28.9113) -> (12.6834, 28.822)
  arc A477 (12.785, 28.6439) -> (12.6834, 28.822) centre (12.6391, 28.6787) ccw
  arc A478 (12.785, 28.6439) -> (12.7614, 28.3231) centre (13.7575, 28.411) ccw
  arc A479 (12.7614, 28.3231) -> (13.115, 27.8542) centre (13.3142, 28.3722) ccw
  arc A480 (13.1024, 27.8603) -> (13.6911, 27.8856) centre (13.3765, 28.3429) ccw
  arc A481 (13.6911, 27.8856) -> (13.9233, 28.1082) centre (13.1243, 28.7095) ccw
  arc A482 (14.1255, 28.1434) -> (13.9233, 28.1082) centre (14.0432, 28.018) ccw
  line L138 (14.3432, 28.0204) -> (14.1255, 28.1434)
  circle A483 centre (0, 0) radius 31.5
  line L139 (10.6099, 29.636) -> (10.8486, 29.5615)
  arc A484 (10.9612, 29.3901) -> (10.8486, 29.5615) centre (10.8134, 29.4157) ccw
  arc A485 (10.9612, 29.3901) -> (10.9578, 29.0685) centre (11.9464, 29.2188) ccw
  arc A486 (10.9578, 29.0685) -> (11.3402, 28.6227) centre (11.5064, 29.1522) ccw
  arc A487 (11.3272, 28.6281) -> (11.9131, 28.6903) centre (11.5705, 29.1269) ccw
  arc A488 (11.9131, 28.6903) -> (12.1309, 28.927) centre (11.2958, 29.477) ccw
  arc A489 (12.3305, 28.9748) -> (12.1309, 28.927) centre (12.2562, 28.8445) ccw
  line L140 (12.5554, 28.8657) -> (12.3305, 28.9748)
  circle A490 centre (0, 0) radius 31.5
  line L141 (8.7281, 30.2437) -> (8.971, 30.1844)
  arc A491 (9.0941, 30.0204) -> (8.971, 30.1844) centre (8.945, 30.0367) ccw
  arc A492 (9.0941, 30.0204) -> (9.1109, 29.6992) centre (10.0882, 29.9113) ccw
  arc A493 (9.1109, 29.6992) -> (9.5206, 29.2783) centre (9.6532, 29.8172) ccw
  arc A494 (9.5073, 29.2828) -> (10.0881, 29.3817) centre (9.7188, 29.7959) ccw
  arc A495 (10.0881, 29.3817) -> (10.2907, 29.6316) centre (9.4226, 30.1281) ccw
  arc A496 (10.4869, 29.6919) -> (10.2907, 29.6316) centre (10.4209, 29.5572) ccw
  line L142 (10.7182, 29.5971) -> (10.4869, 29.6919)
  circle A497 centre (0, 0) radius 31.5
  line L143 (6.8119, 30.732) -> (7.058, 30.6881)
  arc A498 (7.1912, 30.5322) -> (7.058, 30.6881) centre (7.0414, 30.5391) ccw
  arc A499 (7.1912, 30.5322) -> (7.2281, 30.2127) centre (8.1901, 30.4857) ccw
  arc A500 (7.2281, 30.2127) -> (7.6634, 29.8183) centre (7.7619, 30.3645) ccw
  arc A501 (7.6498, 29.822) -> (8.2233, 29.9572) centre (7.8287, 30.3474) ccw
  arc A502 (8.2233, 29.9572) -> (8.4098, 30.2193) centre (7.5122, 30.6603) ccw
  arc A503 (8.6018, 30.2918) -> (8.4098, 30.2193) centre (8.5444, 30.1532) ccw
  line L144 (8.8386, 30.2117) -> (8.6018, 30.2918)
  circle A504 centre (0, 0) radius 31.5
  line L145 (4.8688, 31.0991) -> (5.1172, 31.0708)
  arc A505 (5.2599, 30.9235) -> (5.1172, 31.0708) centre (5.1099, 30.9209) ccw
  arc A506 (5.2599, 30.9235) -> (5.3168, 30.6069) centre (6.2598, 30.9398) ccw
  arc A507 (5.3168, 30.6069) -> (5.776, 30.2407) centre (5.84, 30.792) ccw
  arc A508 (5.7622, 30.2435) -> (6.3261, 30.4144) centre (5.9077, 30.7791) ccw
  arc A509 (6.3261, 30.4144) -> (6.4957, 30.6877) centre (5.5722, 31.0715) ccw
  arc A510 (6.6828, 30.7721) -> (6.4957, 30.6877) centre (6.6342, 30.6302) ccw
  line L146 (6.9242, 30.707) -> (6.6828, 30.7721)
  circle A511 centre (0, 0) radius 31.5
  line L147 (2.9064, 31.3435) -> (3.1561, 31.3308)
  arc A512 (3.3078, 31.1927) -> (3.1561, 31.3308) centre (3.1583, 31.1808) ccw
  arc A513 (3.3078, 31.1927) -> (3.3845, 30.8804) centre (4.3047, 31.2718) ccw
  arc A514 (3.3845, 30.8804) -> (3.8657, 30.5437) centre (3.8951, 31.0979) ccw
  arc A515 (3.8518, 30.5456) -> (4.4039, 30.7516) centre (3.9634, 31.0893) ccw
  arc A516 (4.4039, 30.7516) -> (4.556, 31.035) centre (3.6103, 31.36) ccw
  arc A517 (4.7374, 31.131) -> (4.556, 31.035) centre (4.6978, 30.9863) ccw
  line L148 (4.9824, 31.0812) -> (4.7374, 31.131)
  circle A518 centre (0, 0) radius 31.5
  line L149 (0.9326, 31.4641) -> (1.1826, 31.4671)
  arc A519 (1.3427, 31.3389) -> (1.1826, 31.4671) centre (1.1942, 31.3176) ccw
  arc A520 (1.3427, 31.3389) -> (1.4388, 31.0319) centre (2.3326, 31.4804) ccw
  arc A521 (1.4388, 31.0319) -> (1.9403, 30.7261) centre (1.9347, 31.2811) ccw
  arc A522 (1.9262, 30.7272) -> (2.4643, 30.9675) centre (2.0035, 31.2768) ccw
  arc A523 (2.4643, 30.9675) -> (2.5983, 31.2599) centre (1.634, 31.5248) ccw
  arc A524 (2.7733, 31.367) -> (2.5983, 31.2599) centre (2.7429, 31.2201) ccw
  line L150 (3.021, 31.3327) -> (2.7733, 31.367)
  circle A525 centre (0, 0) radius 31.5
  line L151 (-1.0449, 31.4606) -> (-0.7955, 31.4793)
  arc A526 (-0.6278, 31.3613) -> (-0.7955, 31.4793) centre (-0.7746, 31.3307) ccw
  arc A527 (-0.6278, 31.3613) -> (-0.5126, 31.061) centre (0.3513, 31.5647) ccw
  arc A528 (-0.5126, 31.061) -> (0.0071, 30.7873) centre (-0.0332, 31.3409) ccw
  arc A529 (-0.0069, 30.7875) -> (0.5149, 31.0611) centre (0.0356, 31.3409) ccw
  arc A530 (0.5149, 31.0611) -> (0.6303, 31.3613) centre (-0.3487, 31.5652) ccw
  arc A531 (0.7983, 31.4793) -> (0.6303, 31.3613) centre (0.7772, 31.3308) ccw
  line L152 (1.0476, 31.4606) -> (0.7983, 31.4793)
  circle A532 centre (0, 0) radius 31.5
  line L153 (-3.0182, 31.3329) -> (-2.7706, 31.3672)